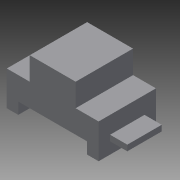
# Autodesk Inventor part: 4.1e Q1
Saved by Autodesk Inventor 2015 (Build 190159000, 159)
## iProperties
Created: 2017-11-13
Part Number: 4.1e Q1
Material: Generic
Document SubType Name: Modeling
Designer: Administrator
Density: 1 g/cm^3
Appearance: Default
Author: Administrator
Autodesk Inventor part; units mm, degrees
ref_plane "YZ Plane" through (0, 0, 0) normal (1, 0, 0) x (0, 1, 0)
ref_plane "XZ Plane" through (0, 0, 0) normal (0, 1, 0) x (-1, 0, 0)
ref_plane "XY Plane" through (0, 0, 0) normal (0, 0, 1) x (1, 0, 0)
sketch "Sketch1" plane through (0, 0, 0) normal (0, 0, 1) x (1, 0, 0)
  line L0 (0, 0) -> (0, 38.1)
  line L1 (0, 38.1) -> (25.4, 38.1)
  line L2 (25.4, 38.1) -> (25.4, 63.5)
  line L3 (25.4, 63.5) -> (76.2, 63.5)
  line L4 (76.2, 63.5) -> (76.2, 38.1)
  line L5 (76.2, 38.1) -> (101.6, 38.1)
  line L6 (101.6, 38.1) -> (101.6, 0)
  line L7 (101.6, 0) -> (88.9, 0)
  line L8 (88.9, 0) -> (88.9, 12.7)
  line L9 (88.9, 12.7) -> (12.7, 12.7)
  line L10 (12.7, 12.7) -> (12.7, 0)
  line L11 (12.7, 0) -> (0, 0)
  dimension "d0" = 38.1
  dimension "d1" = 25.4
  dimension "d2" = 50.8
  dimension "d3" = 76.2
  dimension "d4" = 12.7
  dimension "d5" = 12.7
  dimension "d6" = 12.7
  dimension "d7" = 12.7
  dimension "d8" = 25.4
  constraints: 24 end point, 9 perpendicular, 2 point on line, 2 vertical
  measures "d0" distance of L0.start L0.end
  measures "d1" distance of L0.end L1.end
  measures "d2" distance of L2.end L3.end
  measures "d3" distance of L8.end L9.end
  measures "d4" distance of L9.end L10.end
  measures "d5" distance of L7.end L8.end
  measures "d6" distance of L6.end L7.end
  measures "d7" distance of L10.end L0.start
  measures "d8" distance of L3.end L4.end
extrude "Extrusion1" add sketch "Sketch1" along normal blind 63.5
sketch "Sketch2" plane through (101.6, 0, 0) normal (1, 0, 0) x (0, 0, -1)
  line L0 (-50.8, 19.05) -> (-50.8, 12.7)
  line L1 (0, 12.7) -> (-63.5, 12.7) projected
  line L2 (-12.7, 12.7) -> (-12.7, 19.05)
  line L3 (-12.7, 19.05) -> (-50.8, 19.05)
  point P0 (0, 0)
  dimension "d13" = 38.1
  dimension "d14" = 6.35
  constraints: 6 end point, 2 point on line, 2 vertical, 1 perpendicular
  measures "d13" distance of L2.end L0.start
  measures "d14" distance of L2.start L2.end
extrude "Extrusion2" add sketch "Sketch2" along normal blind 19.05
body "Solid1"
